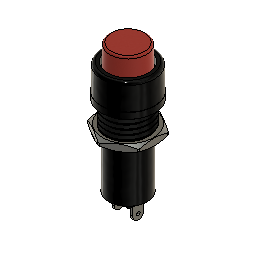
PushButtonSwitch (Autodesk Fusion 360 design; units mm, degrees)
Autodesk Fusion 360 part; units mm, degrees
sketch "Sketch1" plane through (0, 0, 0) normal (0, 0, 1) x (1, 0, 0)
  circle A0 centre (0, 0) radius 5.2
  circle A1 centre (0, 0) radius 6
  circle A2 centre (0, 0) radius 7.2
  circle A3 centre (0, 0) radius 7
  circle A4 centre (0, 0) radius 5.5
  circle A5 centre (0, 0) radius 5.1
  line L0 (-6.95, -4.0126) -> (0, -8.0252)
  line L1 (0, -8.0252) -> (6.95, -4.0126)
  line L2 (6.95, -4.0126) -> (6.95, 4.0126)
  line L3 (6.95, 4.0126) -> (0, 8.0252)
  line L4 (0, 8.0252) -> (-6.95, 4.0126)
  line L5 (-6.95, 4.0126) -> (-6.95, -4.0126)
  dimension "d1" = 10.4
  dimension "d2" = 12
  dimension "d3" = 14.4
  dimension "d4" = 14
  dimension "d5" = 11
  dimension "d19" = 10.2
  dimension "d27" = 6.95
  constraint coincident A0.centre A1.centre
  constraint concentric A0 A1
  constraint concentric A0 A2
  constraint concentric A2 A3
  constraint concentric A2 A4
  constraint concentric A2 A5
  measures "d1" diameter of A0
  measures "d2" diameter of A1
  measures "d3" diameter of A2
  measures "d4" diameter of A3
  measures "d5" diameter of A4
  measures "d19" diameter of A5
  measures "d27" distance of A0.centre L5
extrude "Extrude1" add sketch "Sketch1" against normal blind 14 contours A0 | A5 makes body 1
extrude "Extrude2" add sketch "Sketch1" along normal blind 9.5 contours A0 | A1 | A4 | A5 bodies 1
extrude "Extrude3" add sketch "Sketch1" along normal blind 6.8 from surface at 9.5 contours A1 | A2 A3 L2 | A2 A3 L2 L3 | A2 A3 L1 L2 | A2 A3 L3 | A3 L0 L1 L2 L3 L4 L5 | A3 L2 | A2 A3 L1 | A2 A3 L3 L4 | A3 L3 | A2 A3 L0 L1 | A3 L1 | A2 A3 L4 | A2 A3 L0 | A2 A3 L4 L5 | A3 L4 | A2 A3 L0 L5 | A3 L0 | A2 A3 L5 | A3 L5 bodies 1
thread "Thread1" "ISO Metric profile 12.0 M12x1.25 M12x1.25 6g" major diameter 11.866 minor diameter 10.4385 pitch 1.25 angle 60 modelled right hand crest width 0.1793 on face at (5.9702, -0.5974, 6.3333) crest through (5.933, 0, -0.3125) on bodies 1
chamfer "Chamfer1" distance 0.2 distance2 6.8 1 edges at (-6.7128, -2.6036, 16.3) measured on face at (6.5861, -0.6309, 16.3) on bodies 1
fillet "Fillet1" radius 0.75 1 edges at (-6.5263, 2.5313, 16.3) on bodies 1
extrude "Extrude4" add sketch "Sketch1" along normal blind 11.3 from surface at 9.5 separate body contours A5 makes body 2
chamfer "Chamfer2" distance 0.2 distance2 6 1 edges at (-4.7549, -1.8442, 20.8) measured on face at (-2.0034, -0.5525, 20.8) on bodies 2
fillet "Fillet2" radius 0.5 1 edges at (-4.5684, 1.7719, 20.8) on bodies 2
extrude "Extrude5" add sketch "Sketch1" along normal blind 2 separate body contours A1 | A2 A3 L2 L3 | A2 L2 L3 | A2 L1 L2 | A2 A3 L1 L2 | A3 L0 L1 L2 L3 L4 L5 | A2 A3 L3 L4 | A2 L3 L4 | A2 L0 L1 | A2 A3 L0 L1 | A2 A3 L4 L5 | A2 L4 L5 | A2 L0 L5 | A2 A3 L0 L5 makes body 3
sketch "Sketch2" plane through (0, 0, 0) normal (0, 1, 0) x (1, 0, 0)
  line L0 (0, 0) -> (6.8, 0)
  line L1 (6.8, 0) -> (6.8, -2)
  line L2 (7.9, -1) -> (7.9, -1.325)
  line L3 (7.9, -1.325) -> (6.8, -2)
  line L4 (7.9, -1) -> (7.9, -0.675)
  line L5 (7.9, -0.675) -> (6.8, 0)
  line L6 (6.8, 0) -> (11.8, 0)
  line L7 (11.8, 0) -> (11.8, -2)
  line L8 (11.8, -2) -> (6.8, -2)
  line L9 (6.8, -2) -> (6.8, 0)
  line L10 (0, 0) -> (0, -1)
  line L11 (0, -1) -> (7.9, -1)
  dimension "d30" = 6.8
  dimension "d31" = 0.325
  dimension "d32" = 0.325
  dimension "d33" = 5
  dimension "d34" = 2
  dimension "d35" = 1
  dimension "d36" = 7.9
  dimension "d37" = 2
  constraint coincident L0.start L10.start
  constraint horizontal L0
  constraint perpendicular L0 L1
  constraint horizontal L6
  constraint vertical L7
  constraint horizontal L8
  constraint vertical L9
  constraint perpendicular L0 L10
  constraint perpendicular L10 L11
  constraint coincident L2.start L4.start
  constraint vertical L4
  constraint vertical L2
  measures "d30" distance of L0.start L0.end
  measures "d31" distance of L2.start L2.end
  measures "d32" distance of L2.start L4.end
  measures "d33" distance of L0.end L6.end
  measures "d34" distance of L0.end L1.end
  measures "d35" distance of L0.start L10.end
  measures "d36" distance of L10.end L2.start
  measures "d37" distance of L0.end L1.end
revolve "Revolve1" cut sketch "Sketch2" angle 360 about axis through (0, 0, 1.75) along (0, 0, 1) contours L2 L3 L4 L5 L6 L7 L8 bodies 3
thread "Thread2" "ISO Metric profile 12.0 M12x1.25 M12x1.25 6H" major diameter 12.18 minor diameter 10.7795 pitch 1.25 angle 60 modelled right hand crest width 0.3372 on face at (5.4932, -0.2742, 1.3333) crest through (5.3898, 0, 0.3125) on bodies 3
extrude "Extrude6" add sketch "Sketch1" along normal blind 1.6 separate body contours A1 | A2 A3 L2 | A2 A3 L2 L3 | A2 A3 L1 L2 | A2 A3 L3 | A3 L0 L1 L2 L3 L4 L5 | A3 L2 | A2 A3 L1 | A2 A3 L3 L4 | A3 L3 | A2 A3 L0 L1 | A3 L1 | A2 A3 L4 | A2 A3 L0 | A2 A3 L4 L5 | A3 L4 | A2 A3 L0 L5 | A3 L0 | A2 A3 L5 | A3 L5 makes body 4
move_body "Move1" bodies 4 to x (1, 0, 0) y (0, 1, 0) z (0, 0, 1) at (0, 0, 7)
move_body "Move2" bodies 4 to x (1, 0, 0) y (0, 1, 0) z (0, 0, 1) at (0, 0, 0.8)
move_body "Move3" bodies 3 to x (1, 0, 0) y (0, 1, 0) z (0, 0, 1) at (0, 0, -0.2)
extrude "Extrude7" add 1 faces at (-0.5014, 0.8749, 9.5) along direction (0, 0, 1) blind 1 on bodies 1 bodies 1
extrude "Extrude8" cut 1 faces at (-2.0034, -0.5525, 9.5) along direction (0, 0, 1) blind 1 on bodies 2 bodies 2
sketch "Sketch3" plane through (0, 0, -14) normal (0, 0, -1) x (1, 0, 0)
  circle A0 centre (0, 0) radius 5.2
  line L0 (0, 0) -> (-1.2, 0)
  line L1 (-1.2, 0) -> (-1.2, -3.45)
  line L2 (-1.2, -3.45) -> (-3.8, -3.45)
  line L3 (-3.8, -3.45) -> (-3.8, 3.45)
  line L4 (-3.8, 3.45) -> (-1.2, 3.45)
  line L5 (-1.2, 3.45) -> (-1.2, -3.45)
  line L6 (0, -2.5) -> (0, -20)
  line L7 (1.2, -3.45) -> (3.8, -3.45)
  line L8 (3.8, -3.45) -> (3.8, 3.45)
  line L9 (3.8, 3.45) -> (1.2, 3.45)
  line L10 (1.2, 3.45) -> (1.2, -3.45)
  line L11 (-1.2, 0) -> (-2.5, 0)
  line L12 (-2.8, 2.6) -> (-2.2, 2.6)
  line L13 (-2.2, 2.6) -> (-2.2, -2.6)
  line L14 (-2.2, -2.6) -> (-2.8, -2.6)
  line L15 (-2.8, -2.6) -> (-2.8, 2.6)
  line L16 (-2.8, 2.6) -> (-2.2, -2.6) construction
  line L17 (-2.2, 2.6) -> (-2.8, -2.6) construction
  line L18 (-2.8, 1.5) -> (-2.2, 1.5)
  line L19 (-2.2, 1.5) -> (-2.2, -1.5)
  line L20 (-2.2, -1.5) -> (-2.8, -1.5)
  line L21 (-2.8, -1.5) -> (-2.8, 1.5)
  line L22 (-2.8, 1.5) -> (-2.2, -1.5) construction
  line L23 (-2.2, 1.5) -> (-2.8, -1.5) construction
  line L24 (2.2, -1.5) -> (2.8, -1.5)
  line L25 (2.8, -1.5) -> (2.8, 1.5)
  line L26 (2.8, 1.5) -> (2.2, 1.5)
  line L27 (2.2, 1.5) -> (2.2, -1.5)
  line L28 (2.2, 2.6) -> (2.2, -2.6)
  line L29 (2.2, -2.6) -> (2.8, -2.6)
  line L30 (2.8, 2.6) -> (2.2, 2.6)
  line L31 (2.8, -2.6) -> (2.8, 2.6)
  point P0 (-2.5, 0)
  point P1 (-2.5, 0)
  dimension "d47" = 1.2
  dimension "d48" = 3.45
  dimension "d49" = 2.6
  dimension "d50" = 6.9
  dimension "d54" = 1.3
  dimension "d55" = 0.6
  dimension "d56" = 5.2
  dimension "d57" = 0.6
  dimension "d58" = 3
  constraint coincident A0.centre L0.start
  constraint horizontal L0
  constraint perpendicular L0 L1
  constraint horizontal L2
  constraint vertical L3
  constraint horizontal L4
  constraint vertical L5
  constraint symmetric L1.end L6 L7.start
  constraint symmetric L2.end L6 L7.end
  constraint symmetric L3.end L6 L8.end
  constraint symmetric L4.end L6 L9.end
  constraint perpendicular L3 L11
  constraint horizontal L12
  constraint perpendicular L12 L13
  constraint parallel L12 L14
  constraint parallel L13 L15
  constraint coincident L16 P1
  constraint coincident L17 P1
  constraint coincident P1 P0
  constraint horizontal L18
  constraint perpendicular L18 L19
  constraint parallel L18 L20
  constraint parallel L19 L21
  constraint coincident L22 P1
  constraint coincident L23 P1
  constraint symmetric L6 L12.start L30.start
  constraint symmetric L6 L12.end L28.start
  constraint symmetric L6 L13.end L28.end
  constraint symmetric L6 L14.end L29.end
  constraint symmetric L6 L18.start L25.end
  constraint symmetric L6 L18.end L26.end
  constraint symmetric L6 L19.end L24.start
  constraint symmetric L6 L20.end L24.end
  measures "d47" distance of A0.centre L0.end
  measures "d48" distance of L0.end L1.end
  measures "d49" distance of L1.end L2.end
  measures "d50" distance of L1.end L4.end
  measures "d54" distance of L0.end P1
  measures "d55" distance of L13.end L14.end
  measures "d56" distance of L12.end L13.end
  measures "d57" distance of L19.end L20.end
  measures "d58" distance of L18.end L19.end
extrude "Extrude9" add sketch "Sketch3" along normal blind 0.7 contours L1 L2 L3 L4 L5 | L7 L8 L9 L10 | L12 L13 L15 L18 | L13 L15 L18 L19 L20 L21 | L13 L14 L15 L20 | L24 L25 L26 L27 L28 L31 | L24 L28 L29 L31 | L26 L28 L30 L31 bodies 1
chamfer "Chamfer3" distance 0.5 angle 45 4 edges at (-3.8, 3.45, -14.35) (-3.8, -3.45, -14.35) (3.8, 3.45, -14.35) (3.8, -3.45, -14.35) on bodies 1
extrude "Extrude10" add sketch "Sketch3" along normal blind 0.5 from surface at 0.7 separate body contours L12 L13 L15 L18 | L13 L15 L18 L19 L20 L21 | L13 L14 L15 L20 | L24 L25 L26 L27 L28 L31 | L24 L28 L29 L31 | L26 L28 L30 L31 makes body 5 at (2.4, -0.8667, -14.7) makes body 6 at (-2.6, -0.8667, -14.7)
extrude "Extrude11" add sketch "Sketch3" along normal blind 4.75 from surface at 0.7 contours L13 L15 L18 L19 L20 L21 | L24 L25 L26 L27 L28 L31 bodies 6 makes body 7 at (2.2, -0.5, -17.8667)
fillet "Fillet3" radius 1.5 4 edges at (2.5, -1.5, -19.45) (2.5, 1.5, -19.45) (-2.5, 1.5, -19.45) (-2.5, -1.5, -19.45) on bodies 5 6 7
fillet "Fillet3" radius 0.25 4 edges at (2.5, -2.6, -15.2) (2.5, 2.6, -15.2) (-2.5, -2.6, -15.2) (-2.5, 2.6, -15.2) on bodies 5 6 7
hole "Hole1" at (-2.8, 0, -17.95) direction (1, 0, 0) diameter 1 depth 6 tip angle 118 bodies 6 7
combine "Combine1" operation add target body 7 tool bodies 5
equation "d21 = 6.80 mm + 4.5 mm"
equation "d27 = ( 13.9 / 2 ) * 1 mm"
equation "d30 = ( 13.6 / 2 ) * 1 mm"
equation "d31 = ( 0.65 / 2 ) * 1 mm"
equation "d32 = ( 0.65 / 2 ) * 1 mm"
equation "d36 = ( 15.8 / 2 ) * 1 mm"
equation "d48 = ( 6.9 / 2 ) * 1 mm"
